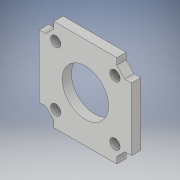
# Autodesk Inventor part: 20_Cube_insert_Sample_holder_magnetic_v3
Saved by Autodesk Inventor 2019 (Build 230136000, 136)
## iProperties
Created: 2020-05-20
Part Number: 20_Cube_insert_Sample_holder_magnetic_v3
Material: Generic
Document SubType Name: Modeling
Designer: B
Density: 1 g/cm^3
Appearance: Default
Author: B
Autodesk Inventor part; units mm, degrees
ref_plane "YZ Plane" through (0, 0, 0) normal (1, 0, 0) x (0, 1, 0)
ref_plane "XZ Plane" through (0, 0, 0) normal (0, 1, 0) x (-1, 0, 0)
ref_plane "XY Plane" through (0, 0, 0) normal (0, 0, 1) x (1, 0, 0)
sketch "Sketch1" plane through (0, 0, 0) normal (0, 0, 1) x (1, 0, 0)
  line L0 (-39.3843, 0) -> (62.0012, 0) construction
  line L1 (0, -36.6008) -> (0, 45.3001) construction
  line L2 (0, 0) -> (33.6, 33.6) construction
  line L3 (0, 0) -> (47.5176, 0) construction
  line L4 (0, 24.9006) -> (16.8, 24.9006)
  line L5 (16.8, 24.9006) -> (16.8, 21.2406)
  line L6 (16.8, 21.2406) -> (19.0203, 19.0203)
  line L7 (24.9006, 0) -> (24.9006, 16.8)
  line L8 (24.9006, 16.8) -> (21.2406, 16.8)
  line L9 (21.2406, 16.8) -> (19.0203, 19.0203)
  line L10 (0, 24.9006) -> (-16.8, 24.9006)
  line L11 (-16.8, 24.9006) -> (-16.8, 21.2406)
  line L12 (-16.8, 21.2406) -> (-19.0203, 19.0203)
  line L13 (-24.9006, 0) -> (-24.9006, 16.8)
  line L14 (-24.9006, 16.8) -> (-21.2406, 16.8)
  line L15 (-21.2406, 16.8) -> (-19.0203, 19.0203)
  line L16 (0, -24.9006) -> (16.8, -24.9006)
  line L17 (16.8, -24.9006) -> (16.8, -21.2406)
  line L18 (16.8, -21.2406) -> (19.0203, -19.0203)
  line L19 (24.9006, 0) -> (24.9006, -16.8)
  line L20 (24.9006, -16.8) -> (21.2406, -16.8)
  line L21 (21.2406, -16.8) -> (19.0203, -19.0203)
  line L22 (0, -24.9006) -> (-16.8, -24.9006)
  line L23 (-16.8, -24.9006) -> (-16.8, -21.2406)
  line L24 (-16.8, -21.2406) -> (-19.0203, -19.0203)
  line L25 (-24.9006, 0) -> (-24.9006, -16.8)
  line L26 (-24.9006, -16.8) -> (-21.2406, -16.8)
  line L27 (-21.2406, -16.8) -> (-19.0203, -19.0203)
  circle A0 centre (0, 0) radius 12.5
  dimension "d0" = 45
  dimension "d1" = 16.8
  dimension "d2" = 3.66
  dimension "d3" = 3.14
  dimension "d4" = 25
  constraints: 52 end point, 20 symmetric about line, 2 horizontal, 2 perpendicular, 2 point on line, 1 centre point, 1 coincident, 1 equal length
  measures "d0" angle of L3 L2
  measures "d1" distance of L4.start L4.end
  measures "d2" distance of L4.end L5.end
  measures "d3" distance of L5.end L6.end
  measures "d4" diameter of A0
extrude "Extrusion1" add sketch "Sketch1" along normal blind 5
sketch "Sketch2" plane through (0, 0, 5) normal (0, 0, 1) x (1, 0, 0)
  circle A0 centre (0, 0) radius 12.5 construction
  line L0 (16.8, 24.9006) -> (-16.8, 24.9006) construction
  line L1 (-16.8, 24.9006) -> (-16.8, 21.2406) construction
  line L2 (-16.8, 21.2406) -> (-21.2406, 16.8) construction
  line L3 (-21.2406, 16.8) -> (-24.9006, 16.8) construction
  line L4 (-24.9006, 16.8) -> (-24.9006, -16.8) construction
  line L5 (-24.9006, -16.8) -> (-21.2406, -16.8) construction
  line L6 (-21.2406, -16.8) -> (-16.8, -21.2406) construction
  line L7 (-16.8, -21.2406) -> (-16.8, -24.9006) construction
  line L8 (-16.8, -24.9006) -> (16.8, -24.9006) construction
  line L9 (16.8, -24.9006) -> (16.8, -21.2406) construction
  line L10 (16.8, -21.2406) -> (21.2406, -16.8) construction
  line L11 (21.2406, -16.8) -> (24.9006, -16.8) construction
  line L12 (24.9006, -16.8) -> (24.9006, 16.8) construction
  line L13 (24.9006, 16.8) -> (21.2406, 16.8) construction
  line L14 (21.2406, 16.8) -> (16.8, 21.2406) construction
  line L15 (16.8, 21.2406) -> (16.8, 24.9006) construction
  circle A1 centre (16.0203, -16.0203) radius 2.1846 construction
  circle A2 centre (-16.0203, -16.0203) radius 2.1846 construction
  circle A3 centre (-16.0203, 16.0203) radius 2.1846 construction
  circle A4 centre (16.0203, 16.0203) radius 2.1846 construction
  circle A5 centre (0, 0) radius 14 construction
  line L16 (-19.0203, 17.0203) -> (-19.0203, -17.0203) construction
  arc A6 (-17.0203, 19.0203) -> (-19.0203, 17.0203) centre (-17.0203, 17.0203) ccw construction
  line L17 (17.0203, 19.0203) -> (-17.0203, 19.0203) construction
  arc A7 (19.0203, 17.0203) -> (17.0203, 19.0203) centre (17.0203, 17.0203) ccw construction
  line L18 (19.0203, -17.0203) -> (19.0203, 17.0203) construction
  arc A8 (17.0203, -19.0203) -> (19.0203, -17.0203) centre (17.0203, -17.0203) ccw construction
  line L19 (-17.0203, -19.0203) -> (17.0203, -19.0203) construction
  arc A9 (-19.0203, -17.0203) -> (-17.0203, -19.0203) centre (-17.0203, -17.0203) ccw construction
  constraints: 4 coincident
hole "Hole1" at (-16.0203, 16.0203, 5) at (16.0203, 16.0203, 5) at (16.0203, -16.0203, 5) at (-16.0203, -16.0203, 5) direction (0, 0, -1) diameter 2.8 end through all counterbore diameter 5.5 counterbore depth 3
sketch "Skizze3" plane through (0, 0, 5) normal (0, 0, 1) x (1, 0, 0)
  circle A0 centre (16.0203, -16.0203) radius 2.75 construction
  circle A1 centre (-16.0203, 16.0203) radius 2.75 construction
  circle A2 centre (16.0203, 16.0203) radius 2.75 construction
  circle A3 centre (-16.0203, -16.0203) radius 2.75 construction
  circle A4 centre (0, 0) radius 12.5 construction
  line L0 (16.8, 24.9006) -> (-16.8, 24.9006) construction
  line L1 (-16.8, 24.9006) -> (-16.8, 21.2406) projected
  line L2 (-16.8, 21.2406) -> (-21.2406, 16.8) projected
  line L3 (-21.2406, 16.8) -> (-24.9006, 16.8) projected
  line L4 (-24.9006, 16.8) -> (-24.9006, -16.8) construction
  line L5 (-24.9006, -16.8) -> (-21.2406, -16.8) projected
  line L6 (-21.2406, -16.8) -> (-16.8, -21.2406) projected
  line L7 (-16.8, -21.2406) -> (-16.8, -24.9006) projected
  line L8 (-16.8, -24.9006) -> (16.8, -24.9006) construction
  line L9 (16.8, -24.9006) -> (16.8, -21.2406) projected
  line L10 (16.8, -21.2406) -> (21.2406, -16.8) projected
  line L11 (21.2406, -16.8) -> (24.9006, -16.8) projected
  line L12 (24.9006, -16.8) -> (24.9006, 16.8) construction
  line L13 (24.9006, 16.8) -> (21.2406, 16.8) projected
  line L14 (21.2406, 16.8) -> (16.8, 21.2406) projected
  line L15 (16.8, 21.2406) -> (16.8, 24.9006) projected
  line L16 (-17, 25.1006) -> (17, 25.1006) construction
  line L17 (17, 25.1006) -> (17, 21.3235)
  line L18 (17, 21.3235) -> (21.3235, 17)
  line L19 (21.3235, 17) -> (25.1006, 17)
  line L20 (25.1006, 17) -> (25.1006, -17) construction
  line L21 (25.1006, -17) -> (21.3235, -17)
  line L22 (21.3235, -17) -> (17, -21.3235)
  line L23 (17, -21.3235) -> (17, -25.1006)
  line L24 (17, -25.1006) -> (-17, -25.1006) construction
  line L25 (-17, -25.1006) -> (-17, -21.3235)
  line L26 (-17, -21.3235) -> (-21.3235, -17)
  line L27 (-21.3235, -17) -> (-25.1006, -17)
  line L28 (-25.1006, -17) -> (-25.1006, 17) construction
  line L29 (-25.1006, 17) -> (-21.3235, 17)
  line L30 (-21.3235, 17) -> (-17, 21.3235)
  line L31 (-17, 21.3235) -> (-17, 25.1006)
  line L32 (-24.9006, 16.8) -> (-24.9006, 17)
  line L33 (-16.8, 24.9006) -> (-17, 24.9006)
  line L34 (16.8, 24.9006) -> (17, 24.9006)
  line L35 (24.9006, 16.8) -> (24.9006, 17)
  line L36 (24.9006, -16.8) -> (24.9006, -17)
  line L37 (16.8, -24.9006) -> (16.8, -21.2406) projected
  line L38 (16.8, -24.9006) -> (17, -24.9006)
  line L39 (-16.8, -24.9006) -> (-17, -24.9006)
  line L40 (-24.9006, -16.8) -> (-24.9006, -17)
  dimension "d14" = 0.2
  constraints: 48 end point, 12 point on line, 3 perpendicular, 1 vertical, 15 other
  measures "d14" distance between parallel lines of L0 L16
extrude "IM_offset" add sketch "Skizze3" against normal up to surface (5 mm away)
body "Solid1"
